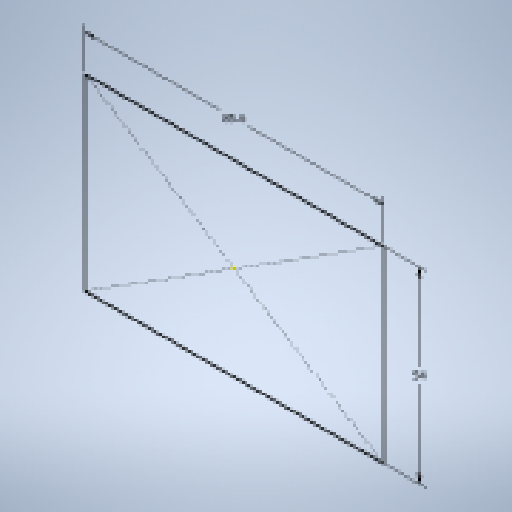
# Autodesk Inventor part: Eazy-Card
Saved by Autodesk Inventor 2023 (Build 270158000, 158)
## iProperties
Created: 2022-04-08
Part Number: Eazy-Card
Material: 一般
Document SubType Name: Modeling
Designer: device
Density: 1 g/cm^3
Appearance: 預設
Author: device
Autodesk Inventor part; units mm, degrees
ref_plane "YZ Plane" through (0, 0, 0) normal (1, 0, 0) x (0, 1, 0)
ref_plane "XZ Plane" through (0, 0, 0) normal (0, 1, 0) x (-1, 0, 0)
ref_plane "XY Plane" through (0, 0, 0) normal (0, 0, 1) x (1, 0, 0)
sketch "草圖1" plane through (0, 0, 0) normal (0, 0, 1) x (1, 0, 0)
  line L0 (-40.8, -27) -> (40.8, -27)
  line L1 (42.8, -25) -> (42.8, 25)
  line L2 (40.8, 27) -> (-40.8, 27)
  line L3 (-42.8, 25) -> (-42.8, -25)
  line L4 (-42.8, -27) -> (42.8, 27) construction
  line L5 (42.8, -27) -> (-42.8, 27) construction
  arc A0 (-40.8, 27) -> (-42.8, 25) centre (-40.8, 25) ccw
  arc A1 (42.8, 25) -> (40.8, 27) centre (40.8, 25) ccw
  arc A2 (40.8, -27) -> (42.8, -25) centre (40.8, -25) ccw
  arc A3 (-42.8, -25) -> (-40.8, -27) centre (-40.8, -25) ccw
  point P0 (0, 0)
  dimension "d0" = 85.6
  dimension "d1" = 54
  dimension "d4" = 2
  constraints: 12 end point, 8 point on circle, 8 point on line, 8 tangent, 4 centre point, 3 equal radius, 2 midpoint, 2 parallel, 1 horizontal, 1 perpendicular
  measures "d0" distance of L5.end L4.end
  measures "d1" distance of L4.end L5.start
  measures "d4" radius of A0
extrude "擠出1" add sketch "草圖1" along normal blind 1
